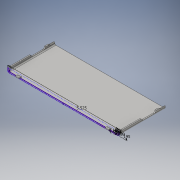
# Autodesk Inventor part: KTR-009
Saved by Autodesk Inventor 2016 (Build 200138000, 138)
## iProperties
Created: 2016-11-11
Part Number: KTR-009
Material: Generic
Document SubType Name: Modeling
Designer: Chris
Density: 1 g/cm^3
Appearance: Default
Author: Chris
Autodesk Inventor part; units mm, degrees
sketch "Sketch1" plane through (0, 0, 0) normal (0, 1, 0) x (-1, 0, 0)
  line L0 (-70.1675, 4.953) -> (70.1675, 4.953) construction
  line L1 (70.1675, 4.953) -> (70.1675, 0) construction
  line L2 (70.1675, 0) -> (-70.1675, 0) construction
  line L3 (-70.1675, 0) -> (-70.1675, 4.953) construction
  line L4 (-67.6275, 0) -> (67.6275, 0)
  arc A0 (67.6275, 0) -> (70.1675, 2.54) centre (67.6275, 2.54) ccw
  line L5 (70.1675, 2.54) -> (70.1675, 4.953)
  arc A1 (-70.1675, 2.54) -> (-67.6275, 0) centre (-67.6275, 2.54) ccw
  line L6 (-70.1675, 2.54) -> (-70.1675, 4.953)
  line L7 (-68.8975, 4.953) -> (-68.8975, 2.54)
  arc A2 (-68.8975, 2.54) -> (-67.6275, 1.27) centre (-67.6275, 2.54) ccw
  line L8 (-67.6275, 1.27) -> (67.6275, 1.27)
  arc A3 (67.6275, 1.27) -> (68.8975, 2.54) centre (67.6275, 2.54) ccw
  line L9 (68.8975, 2.54) -> (68.8975, 4.953)
  line L10 (-70.1675, 4.953) -> (-68.8975, 4.953)
  line L11 (68.8975, 4.953) -> (70.1675, 4.953)
  point P0 (0, 0)
  point P1 (0, 0)
  dimension "d0" = 140.335
  dimension "d1" = 4.953
  dimension "d2" = 1.27
  dimension "d3" = 1.27
  constraints: 24 end point, 8 point on circle, 4 centre point, 4 tangent, 3 equal length, 3 horizontal, 3 horizontal alignment, 3 perpendicular, 2 midpoint, 1 coincident, 1 equal radius, 1 vertical, 4 other
  measures "d0" distance of L0.start L0.end
  measures "d1" distance of L2.end L0.start
  measures "d2" distance between parallel lines of L6 L7
  measures "d3" radius of A2
extrude "Extrusion1" add sketch "Sketch1" along normal blind 58.166
sketch "Sketch2" plane through (-67.6275, 0, 1.27) normal (0, 0, 1) x (1, 0, 0)
  line L0 (-2.54, 0) -> (-2.54, 58.166) projected
  line L1 (137.795, 0) -> (137.795, 58.166) projected
  line L2 (0, 0) -> (135.255, 0) projected
  line L3 (8.89, 2.159) -> (13.3858, 2.159)
  line L4 (13.3858, 2.159) -> (13.3858, -1.524)
  line L5 (13.3858, -1.524) -> (8.89, -1.524)
  line L6 (8.89, -1.524) -> (8.89, 2.159)
  point P0 (67.6275, 0)
  dimension "d6" = 4.4958
  dimension "d7" = 11.43
  dimension "d8" = 3.683
  dimension "d9" = 1.524
  constraints: 8 end point, 2 parallel, 1 horizontal, 1 perpendicular
  measures "d6" distance of L4.end L5.end
  measures "d7" distance between parallel lines of L0 L6
  measures "d8" distance between parallel lines of L5 L3
  measures "d9" distance between parallel lines of L5 L2
extrude "Extrusion2" add sketch "Sketch2" along normal blind 1.016
chamfer "Chamfer2" distance 2.032 distance2 1.016 1 edges at (-56.4896, 2.159, 2.286) measured on face at (-57.2389, 0.9313, 2.286)
sketch "Sketch3" plane through (0, 0, 0) normal (1, 0, 0) x (0, 1, 0)
  line L0 (0, 4.953) -> (58.166, 4.953) projected
  line L1 (0, 2.54) -> (0, 4.953) projected
  line L2 (58.166, 2.54) -> (58.166, 4.953) projected
  line L3 (0, 0) -> (58.166, 0) projected
  line L4 (0, 0) -> (58.166, 0) projected
  line L5 (46.474, 4.953) -> (27.694, 4.953) construction
  line L6 (44.0182, 2.4972) -> (30.1498, 2.4972)
  line L7 (30.1498, 7.4088) -> (44.0182, 7.4088)
  arc A0 (44.0182, 2.4972) -> (44.0182, 7.4088) centre (44.0182, 4.953) ccw
  arc A1 (30.1498, 7.4088) -> (30.1498, 2.4972) centre (30.1498, 4.953) ccw
  line L8 (58.166, 4.0386) -> (52.3421, 4.0386)
  line L9 (51.444, 4.4106) -> (50.9016, 4.953)
  arc A2 (51.444, 4.4106) -> (52.3421, 4.0386) centre (52.3421, 5.3086) ccw
  point P0 (0, 0)
  point P1 (37.084, 4.953)
  point P2 (51.816, 4.0386)
  dimension "d12" = 18.78
  dimension "d13" = 2.4558
  dimension "d15" = 2.4972
  dimension "d16" = 135
  dimension "d17" = 6.35
  dimension "d18" = 0.9144
  dimension "d19" = 1.27
  dimension "d36" = 37.084
  constraints: 12 end point, 8 point on circle, 6 point on line, 6 tangent, 3 centre point, 2 horizontal, 1 collinear, 1 midpoint, 1 parallel
  measures "d12" distance of L5.start L5.end
  measures "d13" distance between parallel lines of L6 L5
  measures "d15" distance between parallel lines of L3 L6
  measures "d16" angle of L8 L9
  measures "d17" distance of L8.start point (51.816, 4.039)
  measures "d18" distance between parallel lines of L0 L8
  measures "d19" radius of A2
  measures "d36" distance from line of point (37.084, 4.953) L1
extrude "Extrusion3" cut sketch "Sketch3" along normal through all both and the other way through all
chamfer "Chamfer1" distance 0.635 angle 45 6 edges at (-68.8975, 55.254, 4.0386) (-68.8975, 51.856, 4.1353) (-68.8975, 51.1728, 4.6818) (68.8975, 55.254, 4.0386) (68.8975, 51.856, 4.1353) (68.8975, 51.1728, 4.6818)
ref_plane "Work Plane1" through (0, 13.97, 0) normal (0, 1, 0) x (-1, 0, 0)
ref_plane "Work Plane2" through (0, 16.51, 0) normal (0, 1, 0) x (-1, 0, 0)
ref_plane "Work Plane3" through (0, 46.99, 0) normal (0, 1, 0) x (-1, 0, 0)
ref_plane "Work Plane4" through (0, 49.53, 0) normal (0, 1, 0) x (-1, 0, 0)
sketch "Sketch6" plane through (0, 0, 0) normal (0, 1, 0) x (-1, 0, 0)
  line L0 (-68.8975, 2.54) -> (-68.8975, 4.953) projected
  arc A0 (-68.8975, 2.54) -> (-67.6275, 1.27) centre (-67.6275, 2.54) ccw projected
  line L1 (-68.8975, 4.953) -> (-68.3895, 4.5009)
  line L2 (-68.3895, 4.5009) -> (-68.8975, 4.0488)
  line L3 (-68.3895, 4.5009) -> (-68.8975, 4.5009) construction
  point P0 (0, 0)
  dimension "d25" = 3.683
  dimension "d26" = 2.7788
  dimension "d27" = 0.508
  constraints: 6 end point, 2 point on line, 1 perpendicular, 1 other
  measures "d25" vertical distance of A0.end L0.end
  measures "d26" vertical distance of A0.end L2.end
  measures "d27" distance of L1.end L3.end
extrude "Extrusion4" add sketch "Sketch6" along normal up to surface (2.54 mm away) from surface at 13.97
extrude "Extrusion5" add sketch "Sketch6" along normal up to surface (2.54 mm away) from surface at 46.99
mirror "Mirror1" about plane through (0, 0, 0) normal (1, 0, 0) of "Extrusion2", "Extrusion4", "Extrusion5", "Chamfer2"
body "Solid1"
